nixal_prusaI3_spoolHolderClear (Autodesk Fusion 360 design; units mm, degrees)
Autodesk Fusion 360 part; units mm, degrees
sketch "Sketch1" plane through (0, 0, 0) normal (0, 1, 0) x (1, 0, 0)
  line L0 (0, 0) -> (30, 0)
  line L1 (30, 0) -> (30, -40)
  line L2 (30, -40) -> (0, -40)
  line L3 (0, -40) -> (0, 0)
  line L4 (0, -40) -> (30, -40)
  line L5 (30, -40) -> (30, -80)
  line L6 (30, -80) -> (0, -80)
  line L7 (0, -80) -> (0, -40)
  line L8 (8, -24) -> (22, -24)
  line L9 (22, -24) -> (22, -32)
  line L10 (22, -32) -> (8, -32)
  line L11 (8, -32) -> (8, -24)
  circle A0 centre (6, -72) radius 2.15
  circle A1 centre (24, -72) radius 2.15
  circle A2 centre (6, -50) radius 2.15
  circle A3 centre (24, -50) radius 2.15
  circle A4 centre (15, -64) radius 4
  circle A5 centre (15, -64) radius 7.5
  dimension "d13" = 14
  dimension "d14" = 8
  dimension "d15" = 8
  dimension "d20" = 40
  dimension "d21" = 4.3
  dimension "d22" = 4.3
  dimension "d23" = 6
  dimension "d24" = 6
  dimension "d27" = 40
  dimension "d28" = 8
  dimension "d32" = 30
  dimension "d33" = 30
  dimension "d45" = 8
  dimension "d46" = 8
  dimension "d47" = 4.3
  dimension "d48" = 4.3
  dimension "d49" = 10
  dimension "d50" = 10
  dimension "d51" = 8
  dimension "d52" = 24
  dimension "d53" = 15
  dimension "d54" = 15
  constraint horizontal L0
  constraint vertical L1
  constraint horizontal L2
  constraint vertical L3
  constraint coincident L0.start L3.end
  constraint horizontal L4
  constraint vertical L5
  constraint horizontal L6
  constraint vertical L7
  constraint horizontal L8
  constraint vertical L9
  constraint horizontal L10
  constraint vertical L11
  constraint concentric A4 A5
  measures "d15" distance of L3 L11
  measures "d21" diameter of A0
  measures "d22" diameter of A1
  measures "d47" diameter of A2
  measures "d48" diameter of A3
  measures "d51" diameter of A4
  measures "d54" diameter of A5
extrude "Extrude1" add sketch "Sketch1" along normal blind 20 contours L0 L1 L2 L3 L4 | L2 L4 L5 L6 L7 | L8 L9 L10 L11 | A0 | A1 | A2 | A3 | A4 | A5
sketch "Sketch2" plane through (30, 0, 0) normal (1, 0, 0) x (0, 0, -1)
  line L0 (-80, 0) -> (0, 0)
  line L1 (0, 0) -> (0, 20)
  line L2 (0, 20) -> (-80, 20)
  line L3 (-80, 20) -> (-80, 0)
  line L4 (-80, 20) -> (-44, 20)
  line L5 (-44, 20) -> (-44, 13.7)
  line L6 (-44, 13.7) -> (-80, 13.7)
  line L7 (-80, 13.7) -> (-80, 20)
  line L8 (-40, 0) -> (-80, 0)
  dimension "d3" = 6.3
  dimension "d43" = 36
  dimension "d44" = 13.7
  constraint horizontal L4
  constraint vertical L5
  constraint horizontal L6
  constraint vertical L7
  constraint coincident L3
  measures "d44" distance of L6 L8
extrude "Extrude2" cut sketch "Sketch2" against normal blind 36 contours L2 L3 L4 L5 L6 L7
sketch "Sketch3" plane through (0, 0, 0) normal (0, 0, -1) x (-1, 0, 0)
  line L0 (-30, 0) -> (0, 0)
  line L1 (0, 0) -> (0, 20)
  line L2 (0, 20) -> (-30, 20)
  line L3 (-30, 20) -> (-30, 0)
  line L4 (-30, 20) -> (0, 0)
  line L5 (0, 20) -> (-30, 0)
  circle A0 centre (-15, 10) radius 4.15
  dimension "d10" = 8.3
  constraint coincident L0.end L1.start
  constraint midpoint L4
  measures "d10" diameter of A0
extrude "Extrude3" cut sketch "Sketch3" against normal blind 40 contours L4 L5 A0 | L4 L5 A0 | L4 L5 A0 | L4 L5 A0
extrude "Extrude4" cut sketch "Sketch1" along normal blind 90 contours L8 L9 L10 L11
extrude "Extrude5" cut sketch "Sketch1" along normal blind 29 contours A0 | A1 | A2 | A3 | A4
extrude "Extrude6" cut sketch "Sketch1" along normal blind 8 and the other way blind 11 contours A5
equation "d1 = DEPTH"
equation "d3 = FRAMETHICKNESS"
equation "d7 = -( FRAMEHIGHT + 8 mm )"
equation "d13 = NUTWINDOWX"
equation "d14 = NUTWINDOWY"
equation "d15 = ( WIDTH - NUTWINDOWX ) / 2"
equation "d20 = FRAMEHIGHT + 12 mm"
equation "d27 = HEIGHTABOVEFRAME"
equation "DEPTH = 20 mm"
equation "FRAMETHICKNESS = 6.3 mm"
equation "WIDTH = 30 mm"
equation "d32 = WIDTH"
equation "d33 = WIDTH"
equation "NUTWINDOWX = 14 mm"
equation "NUTWINDOWY = 8 mm"
equation "HEIGHT = 80 mm"
equation "FRAMEHIGHT = 28 mm" comment "40  for TOP, 28 FOR SIDE"
equation "HEIGHTABOVEFRAME = 40 mm"
equation "d43 = FRAMEHIGHT + 8 mm"
equation "d44 = DEPTH - FRAMETHICKNESS"
